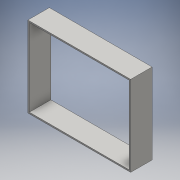
# Autodesk Inventor part: veggur_lok
Saved by Autodesk Inventor 2016 (Build 200138000, 138)
## iProperties
Created: 2016-02-20
Part Number: veggur_lok
Material: Generic
Document SubType Name: Modeling
Designer: Róbert
Density: 1 g/cm^3
Appearance: Default
Author: Róbert
Autodesk Inventor part; units mm, degrees
ref_plane "YZ Plane" through (0, 0, 0) normal (1, 0, 0) x (0, 1, 0)
ref_plane "XZ Plane" through (0, 0, 0) normal (0, 1, 0) x (-1, 0, 0)
ref_plane "XY Plane" through (0, 0, 0) normal (0, 0, 1) x (1, 0, 0)
sketch "Sketch1" plane through (0, 0, 0) normal (0, 1, 0) x (-1, 0, 0)
  line L0 (0, 0) -> (0, -52.5)
  line L1 (0, -52.5) -> (-67.5, -52.5)
  line L2 (-67.5, -52.5) -> (-67.5, 0)
  line L3 (-67.5, 0) -> (0, 0)
  line L4 (-68.5, -53.5) -> (1, -53.5)
  line L5 (1, -53.5) -> (1, 1)
  line L6 (1, 1) -> (-68.5, 1)
  line L7 (-68.5, 1) -> (-68.5, -53.5)
  dimension "d0" = 52.5
  dimension "d1" = 67.5
  dimension "d2" = 52.5
  dimension "d3" = 1
  constraints: 16 end point, 4 perpendicular, 1 vertical, 3 other
  measures "d0" distance of L0.start L0.end
  measures "d1" distance of L0.end L1.end
  measures "d2" distance of L1.end L2.end
  measures "d3" distance between parallel lines of L1 L4
extrude "Extrusion1" add sketch "Sketch1" along normal blind 14.5
body "Solid1"
